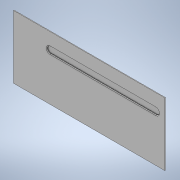
# Autodesk Inventor part: Amb
Saved by Autodesk Inventor 2022 (Build 260153000, 153)
## iProperties
Created: 2022-04-14
Part Number: Amb
Material: Generic
Document SubType Name: Sheet Metal
Designer: Janina
Density: 1 g/cm^3
Sheet Metal Rule: Default_mm
Appearance: Default
Author: Janina
Autodesk Inventor part; units mm, degrees
ref_plane "YZ Plane" through (0, 0, 0) normal (1, 0, 0) x (0, 1, 0)
ref_plane "XZ Plane" through (0, 0, 0) normal (0, 1, 0) x (-1, 0, 0)
ref_plane "XY Plane" through (0, 0, 0) normal (0, 0, 1) x (1, 0, 0)
sketch "Sketch1" plane through (0, 0, 0) normal (0, 0, 1) x (1, 0, 0)
  line L0 (-45, 21.4286) -> (75, 21.4286)
  line L1 (75, 21.4286) -> (75, -28.5714)
  line L2 (75, -28.5714) -> (-45, -28.5714)
  line L3 (-45, -28.5714) -> (-45, 21.4286)
  point P0 (0, 0)
  dimension "d0" = 50
  dimension "d1" = 120
  measures "d0" distance of L0.end L1.end
  measures "d1" distance of L0.start L0.end
extrude "Plate1" add sketch "Sketch1" along normal blind 0.5
sketch "Sketch2" plane through (0, 0, 0.5) normal (0, 0, 1) x (1, 0, 0)
  line L0 (-19.0588, 11.6471) -> (70.9412, 11.6471)
  line L1 (70.9412, 11.6471) -> (70.9412, 5.6471)
  line L2 (70.9412, 5.6471) -> (-19.0588, 5.6471)
  line L3 (-19.0588, 5.6471) -> (-19.0588, 11.6471)
  point P0 (0, 0)
  point P1 (25.9412, 8.6471)
  dimension "LG_A" = 90
  dimension "LT_A" = 6
  dimension "d5" = 45
  dimension "d6" = 3
  constraints: 8 end point, 2 parallel, 1 horizontal, 1 perpendicular
  measures "LG_A" distance of L0.start L0.end
  measures "LT_A" distance of L2.end L0.start
  measures "d5" distance from line of L3 point (25.941, 8.647)
  measures "d6" distance from line of L0 point (25.941, 8.647)
extrude "Extrusion1" add sketch "Sketch2" against normal blind 1.4
sketch "Sketch3" plane through (0, 0, 0.5) normal (0, 0, 1) x (1, 0, 0)
  line L0 (-19.0588, 5.6471) -> (-19.0588, 11.6471) projected
  line L1 (-19.0588, 11.6471) -> (70.9412, 11.6471) projected
  line L2 (70.9412, 11.6471) -> (70.9412, 5.6471) projected
  line L3 (70.9412, 5.6471) -> (-19.0588, 5.6471) projected
  line L4 (-18.5588, 11.1471) -> (70.4412, 11.1471)
  line L5 (70.4412, 11.1471) -> (70.4412, 6.1471)
  line L6 (70.4412, 6.1471) -> (-18.5588, 6.1471)
  line L7 (-18.5588, 6.1471) -> (-18.5588, 11.1471)
  point P0 (0, 0)
  dimension "d9" = 0.5
  dimension "d10" = 0.5
  dimension "d11" = 0.5
  dimension "d12" = 0.5
  constraints: 8 end point, 2 parallel, 1 horizontal, 1 perpendicular
  measures "d9" distance between parallel lines of L1 L4
  measures "d10" distance between parallel lines of L3 L6
  measures "d11" distance between parallel lines of L0 L7
  measures "d12" distance between parallel lines of L2 L5
extrude "Extrusion2" cut sketch "Sketch3" against normal blind 0.9 contours L4 L5 L6 L7
fillet "Fillet1" radius 2.5 4 edges at (-18.5588, 6.1471, 0.05) (-18.5588, 11.1471, 0.05) (70.4412, 11.1471, 0.05) (70.4412, 6.1471, 0.05)
fillet "Fillet2" radius 3 4 edges at (70.9412, 11.6471, -0.45) (70.9412, 5.6471, -0.45) (-19.0588, 11.6471, -0.45) (-19.0588, 5.6471, -0.45)
fillet "Fillet3" radius 0.5 8 edges at (-18.1802, 10.7684, -0.9) (25.9412, 11.6471, -0.9) (70.0625, 10.7684, -0.9) (25.9412, 5.6471, -0.9) (69.709, 10.4149, 0.5) (25.9412, 6.1471, 0.5) (-17.8266, 6.8793, 0.5) (25.9412, 11.1471, 0.5)
fillet "Fillet4" radius 0.2 8 edges at (69.709, 10.4149, -0.4) (25.9412, 6.1471, -0.4) (-17.8266, 6.8793, -0.4) (25.9412, 11.1471, -0.4) (70.0625, 10.7684, 0) (25.9412, 11.6471, 0) (-18.1802, 10.7684, 0) (25.9412, 5.6471, 0)
equation "\"d5\" = 0.5 * LG_A"
equation "\"d6\" = 0.5 * LT_A"
equation "\"d9\" = Thickness"
equation "\"d10\" = Thickness"
equation "\"d11\" = Thickness"
equation "\"d12\" = Thickness"
equation "\"d2\" = Thickness"
equation "\"GapSize\" = Thickness"
equation "\"BendRadius\" = Thickness"
equation "\"MinimumRemnant\" = 2 * Thickness"
equation "\"BendReliefDepth\" = 0.5 * Thickness"
equation "\"BendReliefWidth\" = Thickness"
equation "\"CornerReliefSize\" = 4 * Thickness"
equation "\"JacobiRadiusSize\" = BendRadius"
equation "\"TransitionRadius\" = BendRadius"
equation "\"d15\" = 0.5 * LT_A - Thickness"
equation "\"d16\" = 0.5 * LT_A"
equation "\"d17\" = Thickness"
equation "\"Thickness\" = 0.5"
body "Solid1"
